Autodesk Fusion 360 part; units mm, degrees
(part 4 of 8)
  spline S105 degree 5 poles (194.1162, -114.5953) (194.0941, -114.6123) (193.999, -114.6851) (193.8315, -114.8142) (193.592, -115.0006) (193.2814, -115.2456) (192.9226, -115.5331) (192.5656, -115.8236) (192.2106, -116.117) (191.8576, -116.4134) (191.5064, -116.7127) (191.1571, -117.0147) (190.8096, -117.3193) (190.4637, -117.6264) (190.1196, -117.9359) (189.777, -118.2478) (189.4361, -118.562) (189.0968, -118.8784) (188.759, -119.1971) (188.4229, -119.5179) (188.0883, -119.841) (187.7552, -120.1661) (187.4236, -120.4933) (187.0935, -120.8225) (186.7649, -121.1538) (186.4377, -121.4869) (186.112, -121.822) (185.7877, -122.1589) (185.4648, -122.4977) (185.1433, -122.8384) (184.8232, -123.1808) (184.5045, -123.5251) (184.1871, -123.8711) (183.8711, -124.2188) (183.5565, -124.5682) (183.2431, -124.9194) (182.9312, -125.2722) (182.6205, -125.6266) (182.3112, -125.9826) (182.0031, -126.3403) (181.6964, -126.6995) (181.3909, -127.0603) (181.0867, -127.4227) (180.7838, -127.7866) (180.4822, -128.152) (180.1819, -128.5189) (179.8827, -128.8873) (179.5849, -129.2572) (179.2883, -129.6285) (178.9929, -130.0013) (178.6988, -130.3755) (178.4058, -130.7511) (178.1142, -131.1281) (177.8237, -131.5064) (177.5344, -131.8862) (177.2464, -132.2673) (176.9596, -132.6498) (176.6739, -133.0336) (176.3895, -133.4187) (176.1062, -133.8051) (175.8242, -134.1929) (175.5433, -134.5819) (175.3196, -134.8941) (175.1523, -135.1289) (175.041, -135.2857) (174.9854, -135.3641) knots 0.13851185 0.13851185 0.13851185 0.13851185 0.13851185 0.13851185 0.14285714 0.15714286 0.17142857 0.18571429 0.2 0.21428571 0.22857143 0.24285714 0.25714286 0.27142857 0.28571429 0.3 0.31428571 0.32857143 0.34285714 0.35714286 0.37142857 0.38571429 0.4 0.41428571 0.42857143 0.44285714 0.45714286 0.47142857 0.48571429 0.5 0.51428571 0.52857143 0.54285714 0.55714286 0.57142857 0.58571429 0.6 0.61428571 0.62857143 0.64285714 0.65714286 0.67142857 0.68571429 0.7 0.71428571 0.72857143 0.74285714 0.75714286 0.77142857 0.78571429 0.8 0.81428571 0.82857143 0.84285714 0.85714286 0.87142857 0.88571429 0.9 0.91428571 0.92857143 0.94285714 0.95714286 0.97142857 0.98571429 1 1 1 1 1 1
  arc A53 (174.9854, -135.3641) -> (179.8933, -143.8648) centre (452.3696, 19.1166) ccw
  spline S106 degree 5 poles (179.8933, -143.8648) (179.989, -143.8559) (180.1804, -143.8379) (180.4674, -143.8104) (180.8497, -143.7727) (181.327, -143.724) (181.8038, -143.6736) (182.2801, -143.6215) (182.7558, -143.5677) (183.231, -143.5123) (183.7057, -143.4551) (184.1797, -143.3962) (184.6533, -143.3356) (185.1262, -143.2732) (185.5985, -143.2091) (186.0702, -143.1433) (186.5414, -143.0756) (187.0119, -143.0062) (187.4818, -142.935) (187.951, -142.862) (188.4196, -142.7871) (188.8875, -142.7105) (189.3548, -142.6319) (189.8214, -142.5516) (190.2873, -142.4693) (190.7525, -142.3852) (191.217, -142.2992) (191.6807, -142.2112) (192.1438, -142.1214) (192.606, -142.0295) (193.0676, -141.9357) (193.5283, -141.84) (193.9882, -141.7422) (194.4474, -141.6424) (194.9057, -141.5406) (195.3632, -141.4367) (195.8198, -141.3307) (196.2756, -141.2226) (196.7304, -141.1123) (197.1844, -141) (197.6374, -140.8854) (198.0895, -140.7686) (198.5407, -140.6496) (198.9909, -140.5284) (199.44, -140.4048) (199.8881, -140.2789) (200.3352, -140.1507) (200.7812, -140.02) (201.226, -139.8868) (201.6697, -139.7512) (202.1122, -139.613) (202.5536, -139.4723) (202.9937, -139.329) (203.4326, -139.1831) (203.8702, -139.0344) (204.3064, -138.8829) (204.7411, -138.7284) (205.1743, -138.5708) (205.606, -138.4101) (206.036, -138.2462) (206.4644, -138.0792) (206.8318, -137.9327) (207.113, -137.8185) (207.3086, -137.738) (207.4192, -137.6921) (207.445, -137.6814) knots -1 -1 -1 -1 -1 -1 -0.98571429 -0.97142857 -0.95714286 -0.94285714 -0.92857143 -0.91428571 -0.9 -0.88571429 -0.87142857 -0.85714286 -0.84285714 -0.82857143 -0.81428571 -0.8 -0.78571429 -0.77142857 -0.75714286 -0.74285714 -0.72857143 -0.71428571 -0.7 -0.68571429 -0.67142857 -0.65714286 -0.64285714 -0.62857143 -0.61428571 -0.6 -0.58571429 -0.57142857 -0.55714286 -0.54285714 -0.52857143 -0.51428571 -0.5 -0.48571429 -0.47142857 -0.45714286 -0.44285714 -0.42857143 -0.41428571 -0.4 -0.38571429 -0.37142857 -0.35714286 -0.34285714 -0.32857143 -0.31428571 -0.3 -0.28571429 -0.27142857 -0.25714286 -0.24285714 -0.22857143 -0.21428571 -0.2 -0.18571429 -0.17142857 -0.15714286 -0.14285714 -0.13851185 -0.13851185 -0.13851185 -0.13851185 -0.13851185 -0.13851185
  spline S107 degree 3 poles (209.3868, -138.2841) (209.2745, -138.1106) (209.1293, -137.9607) (208.7896, -137.7251) (208.5983, -137.6415) (208.2383, -137.5621) (208.0756, -137.5516) (207.7528, -137.5802) (207.5946, -137.6192) (207.445, -137.6814) knots 0 0 0 0 0.062015 0.062015 0.12403 0.12403 0.172638 0.172638 0.221247 0.221247 0.221247 0.221247
  arc A54 (209.3868, -138.2841) -> (213.9648, -145.1355) centre (452.3696, 19.1166) ccw
  spline S108 degree 3 poles (213.7785, -147.1602) (213.9249, -147.0143) (214.0414, -146.8411) (214.2013, -146.4599) (214.2433, -146.2555) (214.2463, -145.8867) (214.2227, -145.7255) (214.1277, -145.4157) (214.0567, -145.2689) (213.9648, -145.1355) knots 0 0 0 0 0.062015 0.062015 0.12403 0.12403 0.172638 0.172638 0.221247 0.221247 0.221247 0.221247
  spline S109 degree 5 poles (213.7785, -147.1602) (213.7588, -147.18) (213.6741, -147.2645) (213.5248, -147.4144) (213.3117, -147.6305) (213.0357, -147.9139) (212.7175, -148.2458) (212.4015, -148.5804) (212.0879, -148.9177) (211.7765, -149.2576) (211.4674, -149.6001) (211.1605, -149.9451) (210.8557, -150.2925) (210.5529, -150.6421) (210.2521, -150.9939) (209.9532, -151.3478) (209.6562, -151.7038) (209.3611, -152.0618) (209.0678, -152.4219) (208.7764, -152.7839) (208.4868, -153.1478) (208.199, -153.5136) (207.913, -153.8813) (207.6287, -154.2508) (207.3461, -154.6221) (207.0652, -154.9951) (206.786, -155.3698) (206.5085, -155.7462) (206.2326, -156.1243) (205.9583, -156.504) (205.6856, -156.8853) (205.4145, -157.2682) (205.1451, -157.6526) (204.8772, -158.0386) (204.6108, -158.4262) (204.346, -158.8152) (204.0828, -159.2057) (203.821, -159.5976) (203.5608, -159.991) (203.3021, -160.3858) (203.0448, -160.782) (202.7891, -161.1796) (202.5348, -161.5786) (202.282, -161.9789) (202.0307, -162.3805) (201.7808, -162.7835) (201.5323, -163.1878) (201.2853, -163.5934) (201.0396, -164.0002) (200.7955, -164.4084) (200.5527, -164.8177) (200.3113, -165.2284) (200.0713, -165.6402) (199.8327, -166.0533) (199.5955, -166.4675) (199.3597, -166.883) (199.1252, -167.2996) (198.8921, -167.7174) (198.6604, -168.1364) (198.43, -168.5565) (198.201, -168.9777) (197.9733, -169.4) (197.7922, -169.7388) (197.657, -169.9934) (197.5671, -170.1634) (197.5222, -170.2484) knots 0.13851185 0.13851185 0.13851185 0.13851185 0.13851185 0.13851185 0.14285714 0.15714286 0.17142857 0.18571429 0.2 0.21428571 0.22857143 0.24285714 0.25714286 0.27142857 0.28571429 0.3 0.31428571 0.32857143 0.34285714 0.35714286 0.37142857 0.38571429 0.4 0.41428571 0.42857143 0.44285714 0.45714286 0.47142857 0.48571429 0.5 0.51428571 0.52857143 0.54285714 0.55714286 0.57142857 0.58571429 0.6 0.61428571 0.62857143 0.64285714 0.65714286 0.67142857 0.68571429 0.7 0.71428571 0.72857143 0.74285714 0.75714286 0.77142857 0.78571429 0.8 0.81428571 0.82857143 0.84285714 0.85714286 0.87142857 0.88571429 0.9 0.91428571 0.92857143 0.94285714 0.95714286 0.97142857 0.98571429 1 1 1 1 1 1
  arc A55 (197.5222, -170.2484) -> (203.4977, -178.0357) centre (452.3696, 19.1166) ccw
  spline S110 degree 5 poles (203.4977, -178.0357) (203.5914, -178.0144) (203.7789, -177.9716) (204.0598, -177.9069) (204.4339, -177.8197) (204.9008, -177.709) (205.3669, -177.5968) (205.8323, -177.483) (206.297, -177.3676) (206.7609, -177.2506) (207.224, -177.132) (207.6863, -177.0117) (208.1479, -176.8898) (208.6086, -176.7662) (209.0685, -176.641) (209.5276, -176.5141) (209.9859, -176.3856) (210.4433, -176.2553) (210.8999, -176.1234) (211.3556, -175.9898) (211.8104, -175.8544) (212.2643, -175.7173) (212.7173, -175.5785) (213.1695, -175.4379) (213.6206, -175.2955) (214.0709, -175.1514) (214.5202, -175.0055) (214.9685, -174.8578) (215.4158, -174.7082) (215.8621, -174.5568) (216.3075, -174.4036) (216.7518, -174.2485) (217.195, -174.0916) (217.6372, -173.9327) (218.0783, -173.7719) (218.5183, -173.6092) (218.9572, -173.4445) (219.3949, -173.2778) (219.8315, -173.1092) (220.2669, -172.9385) (220.7012, -172.7658) (221.1341, -172.591) (221.5659, -172.4141) (221.9964, -172.2352) (222.4256, -172.054) (222.8534, -171.8707) (223.2799, -171.6852) (223.705, -171.4974) (224.1287, -171.3073) (224.5509, -171.1149) (224.9716, -170.9202) (225.3908, -170.7231) (225.8085, -170.5236) (226.2246, -170.3216) (226.639, -170.1171) (227.0517, -169.9099) (227.4625, -169.7) (227.8715, -169.4872) (228.2784, -169.2716) (228.6834, -169.053) (229.0863, -168.8315) (229.4315, -168.6383) (229.6954, -168.4883) (229.8788, -168.3829) (229.9824, -168.323) (230.0066, -168.309) knots -1 -1 -1 -1 -1 -1 -0.98571429 -0.97142857 -0.95714286 -0.94285714 -0.92857143 -0.91428571 -0.9 -0.88571429 -0.87142857 -0.85714286 -0.84285714 -0.82857143 -0.81428571 -0.8 -0.78571429 -0.77142857 -0.75714286 -0.74285714 -0.72857143 -0.71428571 -0.7 -0.68571429 -0.67142857 -0.65714286 -0.64285714 -0.62857143 -0.61428571 -0.6 -0.58571429 -0.57142857 -0.55714286 -0.54285714 -0.52857143 -0.51428571 -0.5 -0.48571429 -0.47142857 -0.45714286 -0.44285714 -0.42857143 -0.41428571 -0.4 -0.38571429 -0.37142857 -0.35714286 -0.34285714 -0.32857143 -0.31428571 -0.3 -0.28571429 -0.27142857 -0.25714286 -0.24285714 -0.22857143 -0.21428571 -0.2 -0.18571429 -0.17142857 -0.15714286 -0.14285714 -0.13851185 -0.13851185 -0.13851185 -0.13851185 -0.13851185 -0.13851185
  spline S111 degree 3 poles (232.0105, -168.6531) (231.8764, -168.4958) (231.7129, -168.3662) (231.3454, -168.1768) (231.1449, -168.119) (230.7775, -168.0872) (230.6149, -168.098) (230.2986, -168.1686) (230.1468, -168.2278) (230.0066, -168.309) knots 0 0 0 0 0.062015 0.062015 0.12403 0.12403 0.172638 0.172638 0.221247 0.221247 0.221247 0.221247
  arc A56 (232.0105, -168.6531) -> (237.4436, -174.8484) centre (452.3696, 19.1166) ccw
  spline S112 degree 3 poles (237.5232, -176.8801) (237.6493, -176.7163) (237.7421, -176.5294) (237.851, -176.1305) (237.8659, -175.9224) (237.8207, -175.5564) (237.7763, -175.3996) (237.6417, -175.1049) (237.5521, -174.9687) (237.4436, -174.8484) knots 0 0 0 0 0.062015 0.062015 0.12403 0.12403 0.172638 0.172638 0.221247 0.221247 0.221247 0.221247
  spline S113 degree 5 poles (237.5232, -176.8801) (237.5062, -176.9022) (237.4332, -176.9971) (237.3048, -177.1652) (237.1217, -177.4073) (236.8851, -177.7243) (236.6129, -178.0949) (236.3433, -178.4678) (236.0764, -178.8431) (235.8121, -179.2208) (235.5503, -179.6007) (235.2911, -179.9829) (235.0342, -180.367) (234.7796, -180.7532) (234.5273, -181.1413) (234.2772, -181.5312) (234.0292, -181.9229) (233.7833, -182.3164) (233.5396, -182.7116) (233.2979, -183.1085) (233.0583, -183.5071) (232.8207, -183.9074) (232.5851, -184.3093) (232.3515, -184.7127) (232.1198, -185.1177) (231.89, -185.5242) (231.6621, -185.9321) (231.436, -186.3415) (231.2118, -186.7524) (230.9894, -187.1646) (230.7689, -187.5783) (230.5501, -187.9933) (230.3331, -188.4096) (230.1179, -188.8273) (229.9044, -189.2463) (229.6927, -189.6665) (229.4826, -190.088) (229.2743, -190.5108) (229.0676, -190.9347) (228.8626, -191.3599) (228.6593, -191.7863) (228.4577, -192.2139) (228.2576, -192.6427) (228.0592, -193.0726) (227.8625, -193.5036) (227.6673, -193.9357) (227.4737, -194.369) (227.2818, -194.8033) (227.0914, -195.2388) (226.9025, -195.6753) (226.7152, -196.1129) (226.5295, -196.5515) (226.3454, -196.9911) (226.1627, -197.4318) (225.9816, -197.8735) (225.802, -198.3162) (225.624, -198.7598) (225.4474, -199.2045) (225.2723, -199.6501) (225.0987, -200.0967) (224.9266, -200.5442) (224.756, -200.9926) (224.6207, -201.3522) (224.5199, -201.6222) (224.453, -201.8024) (224.4196, -201.8926) knots 0.13851185 0.13851185 0.13851185 0.13851185 0.13851185 0.13851185 0.14285714 0.15714286 0.17142857 0.18571429 0.2 0.21428571 0.22857143 0.24285714 0.25714286 0.27142857 0.28571429 0.3 0.31428571 0.32857143 0.34285714 0.35714286 0.37142857 0.38571429 0.4 0.41428571 0.42857143 0.44285714 0.45714286 0.47142857 0.48571429 0.5 0.51428571 0.52857143 0.54285714 0.55714286 0.57142857 0.58571429 0.6 0.61428571 0.62857143 0.64285714 0.65714286 0.67142857 0.68571429 0.7 0.71428571 0.72857143 0.74285714 0.75714286 0.77142857 0.78571429 0.8 0.81428571 0.82857143 0.84285714 0.85714286 0.87142857 0.88571429 0.9 0.91428571 0.92857143 0.94285714 0.95714286 0.97142857 0.98571429 1 1 1 1 1 1
  arc A57 (224.4196, -201.8926) -> (231.3604, -208.8334) centre (452.3696, 19.1166) ccw
  spline S114 degree 5 poles (231.3604, -208.8334) (231.4505, -208.8) (231.6307, -208.7331) (231.9008, -208.6323) (232.2603, -208.4969) (232.7088, -208.3263) (233.1563, -208.1542) (233.6029, -207.9807) (234.0485, -207.8056) (234.4931, -207.629) (234.9368, -207.4509) (235.3795, -207.2713) (235.8212, -207.0902) (236.2619, -206.9076) (236.7015, -206.7234) (237.1401, -206.5377) (237.5777, -206.3504) (238.0142, -206.1616) (238.4496, -205.9712) (238.884, -205.7792) (239.3172, -205.5857) (239.7494, -205.3905) (240.1804, -205.1937) (240.6103, -204.9953) (241.039, -204.7953) (241.4666, -204.5936) (241.893, -204.3903) (242.3182, -204.1853) (242.7422, -203.9787) (243.165, -203.7704) (243.5865, -203.5603) (244.0067, -203.3486) (244.4257, -203.1351) (244.8433, -202.9198) (245.2597, -202.7029) (245.6747, -202.4841) (246.0883, -202.2635) (246.5006, -202.0412) (246.9114, -201.817) (247.3208, -201.5909) (247.7288, -201.363) (248.1353, -201.1332) (248.5402, -200.9015) (248.9437, -200.6678) (249.3456, -200.4323) (249.7458, -200.1947) (250.1445, -199.9551) (250.5414, -199.7134) (250.9366, -199.4696) (251.3301, -199.2238) (251.7218, -198.9758) (252.1117, -198.7256) (252.4997, -198.4733) (252.8859, -198.2188) (253.2701, -197.9619) (253.6522, -197.7027) (254.0322, -197.4409) (254.4098, -197.1766) (254.7851, -196.9096) (255.1581, -196.6401) (255.5287, -196.3678) (255.8457, -196.1313) (256.0877, -195.9482) (256.2558, -195.8197) (256.3507, -195.7468) (256.3729, -195.7298) knots -1 -1 -1 -1 -1 -1 -0.98571429 -0.97142857 -0.95714286 -0.94285714 -0.92857143 -0.91428571 -0.9 -0.88571429 -0.87142857 -0.85714286 -0.84285714 -0.82857143 -0.81428571 -0.8 -0.78571429 -0.77142857 -0.75714286 -0.74285714 -0.72857143 -0.71428571 -0.7 -0.68571429 -0.67142857 -0.65714286 -0.64285714 -0.62857143 -0.61428571 -0.6 -0.58571429 -0.57142857 -0.55714286 -0.54285714 -0.52857143 -0.51428571 -0.5 -0.48571429 -0.47142857 -0.45714286 -0.44285714 -0.42857143 -0.41428571 -0.4 -0.38571429 -0.37142857 -0.35714286 -0.34285714 -0.32857143 -0.31428571 -0.3 -0.28571429 -0.27142857 -0.25714286 -0.24285714 -0.22857143 -0.21428571 -0.2 -0.18571429 -0.17142857 -0.15714286 -0.14285714 -0.13851185 -0.13851185 -0.13851185 -0.13851185 -0.13851185 -0.13851185
  spline S115 degree 3 poles (258.4046, -195.8094) (258.2511, -195.6709) (258.0721, -195.5637) (257.683, -195.424) (257.4766, -195.3928) (257.1083, -195.4092) (256.9484, -195.4412) (256.6441, -195.5524) (256.5013, -195.631) (256.3729, -195.7298) knots 0 0 0 0 0.062015 0.062015 0.12403 0.12403 0.172638 0.172638 0.221247 0.221247 0.221247 0.221247
  arc A58 (258.4046, -195.8094) -> (264.5998, -201.2425) centre (452.3696, 19.1166) ccw
  spline S116 degree 3 poles (264.9439, -203.2464) (265.0475, -203.0675) (265.1152, -202.8701) (265.1711, -202.4605) (265.1587, -202.2522) (265.0661, -201.8952) (265.0017, -201.7455) (264.8297, -201.4709) (264.7232, -201.3475) (264.5998, -201.2425) knots 0 0 0 0 0.062015 0.062015 0.12403 0.12403 0.172638 0.172638 0.221247 0.221247 0.221247 0.221247
  spline S117 degree 5 poles (264.9439, -203.2464) (264.9299, -203.2706) (264.87, -203.3742) (264.7646, -203.5576) (264.6147, -203.8215) (264.4215, -204.1666) (264.2, -204.5696) (263.9814, -204.9746) (263.7657, -205.3815) (263.553, -205.7904) (263.343, -206.2013) (263.1359, -206.614) (262.9314, -207.0284) (262.7294, -207.4445) (262.5299, -207.8622) (262.3328, -208.2814) (262.138, -208.7021) (261.9456, -209.1243) (261.7555, -209.5479) (261.5678, -209.973) (261.3822, -210.3995) (261.1989, -210.8274) (261.0178, -211.2566) (260.8388, -211.6871) (260.662, -212.1188) (260.4872, -212.5518) (260.3145, -212.986) (260.1438, -213.4214) (259.9751, -213.858) (259.8085, -214.2958) (259.6438, -214.7347) (259.4811, -215.1747) (259.3203, -215.6158) (259.1614, -216.058) (259.0044, -216.5012) (258.8493, -216.9455) (258.6961, -217.3908) (258.5447, -217.8372) (258.3952, -218.2845) (258.2475, -218.7328) (258.1016, -219.1821) (257.9574, -219.6323) (257.8151, -220.0835) (257.6745, -220.5356) (257.5357, -220.9886) (257.3986, -221.4426) (257.2632, -221.8974) (257.1296, -222.3531) (256.9976, -222.8097) (256.8674, -223.2671) (256.7388, -223.7253) (256.612, -224.1844) (256.4867, -224.6444) (256.3632, -225.1051) (256.2413, -225.5666) (256.121, -226.029) (256.0024, -226.4921) (255.8854, -226.956) (255.7699, -227.4206) (255.6561, -227.8861) (255.5439, -228.3522) (255.4333, -228.8191) (255.3461, -229.1932) (255.2814, -229.4741) (255.2386, -229.6615) (255.2172, -229.7553) knots 0.13851185 0.13851185 0.13851185 0.13851185 0.13851185 0.13851185 0.14285714 0.15714286 0.17142857 0.18571429 0.2 0.21428571 0.22857143 0.24285714 0.25714286 0.27142857 0.28571429 0.3 0.31428571 0.32857143 0.34285714 0.35714286 0.37142857 0.38571429 0.4 0.41428571 0.42857143 0.44285714 0.45714286 0.47142857 0.48571429 0.5 0.51428571 0.52857143 0.54285714 0.55714286 0.57142857 0.58571429 0.6 0.61428571 0.62857143 0.64285714 0.65714286 0.67142857 0.68571429 0.7 0.71428571 0.72857143 0.74285714 0.75714286 0.77142857 0.78571429 0.8 0.81428571 0.82857143 0.84285714 0.85714286 0.87142857 0.88571429 0.9 0.91428571 0.92857143 0.94285714 0.95714286 0.97142857 0.98571429 1 1 1 1 1 1
  arc A59 (255.2172, -229.7553) -> (263.0046, -235.7307) centre (452.3696, 19.1166) ccw
  spline S118 degree 5 poles (263.0046, -235.7307) (263.0896, -235.6859) (263.2595, -235.596) (263.5141, -235.4608) (263.8529, -235.2797) (264.2753, -235.052) (264.6965, -234.823) (265.1166, -234.5926) (265.5355, -234.3608) (265.9533, -234.1277) (266.37, -233.8933) (266.7854, -233.6575) (267.1997, -233.4202) (267.6128, -233.1817) (268.0246, -232.9417) (268.4352, -232.7003) (268.8446, -232.4575) (269.2527, -232.2133) (269.6596, -231.9677) (270.0652, -231.7207) (270.4695, -231.4722) (270.8724, -231.2223) (271.2741, -230.971) (271.6744, -230.7181) (272.0734, -230.4639) (272.471, -230.2081) (272.8672, -229.9509) (273.262, -229.6922) (273.6554, -229.4319) (274.0473, -229.1702) (274.4378, -228.9069) (274.8268, -228.6421) (275.2143, -228.3758) (275.6003, -228.1079) (275.9848, -227.8384) (276.3677, -227.5674) (276.749, -227.2947) (277.1287, -227.0204) (277.5068, -226.7445) (277.8832, -226.4669) (278.2579, -226.1877) (278.6309, -225.9068) (279.0021, -225.6243) (279.3716, -225.34) (279.7393, -225.0539) (280.1052, -224.7661) (280.4691, -224.4766) (280.8311, -224.1851) (281.1911, -223.8919) (281.5491, -223.5968) (281.9051, -223.2998) (282.259, -223.0009) (282.6108, -222.7001) (282.9605, -222.3973) (283.3079, -222.0925) (283.6529, -221.7856) (283.9954, -221.4765) (284.3353, -221.1651) (284.6726, -220.8515) (285.0071, -220.5355) (285.3391, -220.2172) (285.6225, -219.9413) (285.8385, -219.7282) (285.9884, -219.5789) (286.073, -219.4942) (286.0927, -219.4744) knots -1 -1 -1 -1 -1 -1 -0.98571429 -0.97142857 -0.95714286 -0.94285714 -0.92857143 -0.91428571 -0.9 -0.88571429 -0.87142857 -0.85714286 -0.84285714 -0.82857143 -0.81428571 -0.8 -0.78571429 -0.77142857 -0.75714286 -0.74285714 -0.72857143 -0.71428571 -0.7 -0.68571429 -0.67142857 -0.65714286 -0.64285714 -0.62857143 -0.61428571 -0.6 -0.58571429 -0.57142857 -0.55714286 -0.54285714 -0.52857143 -0.51428571 -0.5 -0.48571429 -0.47142857 -0.45714286 -0.44285714 -0.42857143 -0.41428571 -0.4 -0.38571429 -0.37142857 -0.35714286 -0.34285714 -0.32857143 -0.31428571 -0.3 -0.28571429 -0.27142857 -0.25714286 -0.24285714 -0.22857143 -0.21428571 -0.2 -0.18571429 -0.17142857 -0.15714286 -0.14285714 -0.13851185 -0.13851185 -0.13851185 -0.13851185 -0.13851185 -0.13851185
  spline S119 degree 3 poles (288.1174, -219.2882) (287.9472, -219.1709) (287.7557, -219.088) (287.3517, -219.0002) (287.1431, -218.9962) (286.78, -219.0606) (286.6257, -219.1132) (286.3384, -219.2632) (286.2071, -219.3597) (286.0927, -219.4744) knots 0 0 0 0 0.062015 0.062015 0.12403 0.12403 0.172638 0.172638 0.221247 0.221247 0.221247 0.221247
  arc A60 (288.1174, -219.2882) -> (294.9688, -223.8661) centre (452.3696, 19.1166) ccw
  spline S120 degree 3 poles (295.5716, -225.808) (295.6509, -225.6171) (295.6923, -225.4126) (295.6942, -224.9992) (295.6548, -224.7942) (295.5164, -224.4524) (295.4329, -224.3125) (295.2265, -224.0626) (295.1048, -223.9542) (294.9688, -223.8661) knots 0 0 0 0 0.062015 0.062015 0.12403 0.12403 0.172638 0.172638 0.221247 0.221247 0.221247 0.221247
  spline S121 degree 5 poles (295.5716, -225.808) (295.5609, -225.8338) (295.515, -225.9443) (295.4344, -226.14) (295.3202, -226.4211) (295.1737, -226.7886) (295.0067, -227.217) (294.8429, -227.647) (294.6821, -228.0786) (294.5246, -228.5118) (294.3701, -228.9466) (294.2186, -229.3828) (294.0699, -229.8203) (293.924, -230.2592) (293.7807, -230.6994) (293.64, -231.1407) (293.5018, -231.5833) (293.3661, -232.027) (293.233, -232.4718) (293.1023, -232.9178) (292.974, -233.3648) (292.8481, -233.813) (292.7246, -234.2621) (292.6033, -234.7123) (292.4843, -235.1634) (292.3676, -235.6155) (292.253, -236.0686) (292.1406, -236.5225) (292.0304, -236.9774) (291.9223, -237.4332) (291.8163, -237.8898) (291.7124, -238.3473) (291.6106, -238.8056) (291.5108, -239.2647) (291.413, -239.7247) (291.3172, -240.1854) (291.2234, -240.6469) (291.1316, -241.1092) (291.0417, -241.5722) (290.9538, -242.036) (290.8678, -242.5005) (290.7836, -242.9657) (290.7014, -243.4316) (290.621, -243.8982) (290.5425, -244.3654) (290.4658, -244.8334) (290.391, -245.302) (290.318, -245.7712) (290.2468, -246.2411) (290.1774, -246.7116) (290.1097, -247.1827) (290.0438, -247.6545) (289.9797, -248.1268) (289.9174, -248.5997) (289.8568, -249.0732) (289.7979, -249.5473) (289.7407, -250.0219) (289.6852, -250.4971) (289.6314, -250.9729) (289.5794, -251.4492) (289.529, -251.926) (289.4802, -252.4033) (289.4426, -252.7856) (289.4151, -253.0726) (289.3971, -253.264) (289.3882, -253.3597) knots 0.13851185 0.13851185 0.13851185 0.13851185 0.13851185 0.13851185 0.14285714 0.15714286 0.17142857 0.18571429 0.2 0.21428571 0.22857143 0.24285714 0.25714286 0.27142857 0.28571429 0.3 0.31428571 0.32857143 0.34285714 0.35714286 0.37142857 0.38571429 0.4 0.41428571 0.42857143 0.44285714 0.45714286 0.47142857 0.48571429 0.5 0.51428571 0.52857143 0.54285714 0.55714286 0.57142857 0.58571429 0.6 0.61428571 0.62857143 0.64285714 0.65714286 0.67142857 0.68571429 0.7 0.71428571 0.72857143 0.74285714 0.75714286 0.77142857 0.78571429 0.8 0.81428571 0.82857143 0.84285714 0.85714286 0.87142857 0.88571429 0.9 0.91428571 0.92857143 0.94285714 0.95714286 0.97142857 0.98571429 1 1 1 1 1 1
  arc A61 (289.3882, -253.3597) -> (297.8889, -258.2676) centre (452.3696, 19.1166) ccw
  spline S122 degree 5 poles (297.8889, -258.2676) (297.9673, -258.212) (298.1241, -258.1007) (298.3588, -257.9334) (298.6711, -257.7097) (299.0601, -257.4288) (299.4478, -257.1467) (299.8343, -256.8635) (300.2194, -256.579) (300.6032, -256.2934) (300.9856, -256.0066) (301.3668, -255.7185) (301.7465, -255.4293) (302.1249, -255.1388) (302.5019, -254.8471) (302.8775, -254.5542) (303.2517, -254.2601) (303.6245, -253.9647) (303.9958, -253.6681) (304.3656, -253.3702) (304.734, -253.0711) (305.1009, -252.7707) (305.4664, -252.4691) (305.8303, -252.1662) (306.1926, -251.8621) (306.5534, -251.5566) (306.9127, -251.2498) (307.2703, -250.9418) (307.6264, -250.6325) (307.9808, -250.3218) (308.3336, -250.0098) (308.6847, -249.6965) (309.0342, -249.3819) (309.3819, -249.0659) (309.7279, -248.7485) (310.0721, -248.4298) (310.4146, -248.1097) (310.7552, -247.7882) (311.094, -247.4653) (311.431, -247.141) (311.7661, -246.8153) (312.0992, -246.4881) (312.4304, -246.1595) (312.7596, -245.8294) (313.0869, -245.4978) (313.412, -245.1647) (313.735, -244.8301) (314.0559, -244.4939) (314.3746, -244.1562) (314.691, -243.8169) (315.0051, -243.4759) (315.317, -243.1334) (315.6266, -242.7892) (315.9337, -242.4434) (316.2383, -242.0959) (316.5403, -241.7465) (316.8396, -241.3954) (317.1359, -241.0423) (317.4294, -240.6873) (317.7198, -240.3304) (318.0074, -239.9716) (318.2523, -239.661) (318.4387, -239.4215) (318.5679, -239.2539) (318.6407, -239.1589) (318.6576, -239.1367) knots -1 -1 -1 -1 -1 -1 -0.98571429 -0.97142857 -0.95714286 -0.94285714 -0.92857143 -0.91428571 -0.9 -0.88571429 -0.87142857 -0.85714286 -0.84285714 -0.82857143 -0.81428571 -0.8 -0.78571429 -0.77142857 -0.75714286 -0.74285714 -0.72857143 -0.71428571 -0.7 -0.68571429 -0.67142857 -0.65714286 -0.64285714 -0.62857143 -0.61428571 -0.6 -0.58571429 -0.57142857 -0.55714286 -0.54285714 -0.52857143 -0.51428571 -0.5 -0.48571429 -0.47142857 -0.45714286 -0.44285714 -0.42857143 -0.41428571 -0.4 -0.38571429 -0.37142857 -0.35714286 -0.34285714 -0.32857143 -0.31428571 -0.3 -0.28571429 -0.27142857 -0.25714286 -0.24285714 -0.22857143 -0.21428571 -0.2 -0.18571429 -0.17142857 -0.15714286 -0.14285714 -0.13851185 -0.13851185 -0.13851185 -0.13851185 -0.13851185 -0.13851185
  spline S123 degree 3 poles (320.6407, -238.6878) (320.4566, -238.5937) (320.2559, -238.5365) (319.8439, -238.5023) (319.6366, -238.5255) (319.285, -238.6368) (319.1389, -238.709) (318.8737, -238.8952) (318.7561, -239.0081) (318.6576, -239.1367) knots 0 0 0 0 0.062015 0.062015 0.12403 0.12403 0.172638 0.172638 0.221247 0.221247 0.221247 0.221247
  arc A62 (320.6407, -238.6878) -> (328.031, -242.3323) centre (452.3696, 19.1166) ccw
  spline S124 degree 3 poles (328.8821, -244.1789) (328.9359, -243.9793) (328.9501, -243.7711) (328.8981, -243.3609) (328.8322, -243.1629) (328.6504, -242.8421) (328.5494, -242.7142) (328.3122, -242.4935) (328.1774, -242.4019) (328.031, -242.3323) knots 0 0 0 0 0.062015 0.062015 0.12403 0.12403 0.172638 0.172638 0.221247 0.221247 0.221247 0.221247
  spline S125 degree 5 poles (328.8821, -244.1789) (328.8748, -244.2058) (328.8438, -244.3214) (328.7894, -244.5259) (328.7129, -244.8196) (328.6156, -245.203) (328.506, -245.6495) (328.3996, -246.0973) (328.2966, -246.5462) (328.1969, -246.9962) (328.1005, -247.4474) (328.0072, -247.8997) (327.9169, -248.3529) (327.8296, -248.8071) (327.7449, -249.2622) (327.663, -249.7181) (327.5838, -250.1749) (327.5073, -250.6325) (327.4333, -251.0909) (327.3619, -251.5501) (327.2931, -252.0101) (327.2268, -252.4708) (327.1629, -252.9323) (327.1015, -253.3944) (327.0424, -253.8572) (326.9856, -254.3207) (326.9312, -254.7848) (326.879, -255.2496) (326.8291, -255.7149) (326.7814, -256.1809) (326.7359, -256.6475) (326.6926, -257.1146) (326.6515, -257.5823) (326.6125, -258.0505) (326.5756, -258.5193) (326.5408, -258.9886) (326.508, -259.4584) (326.4773, -259.9287) (326.4486, -260.3995) (326.422, -260.8708) (326.3973, -261.3425) (326.3746, -261.8147) (326.3539, -262.2874) (326.3351, -262.7605) (326.3183, -263.234) (326.3033, -263.7079) (326.2903, -264.1823) (326.2792, -264.657) (326.2699, -265.1322) (326.2625, -265.6077) (326.2569, -266.0837) (326.2532, -266.5599) (326.2513, -267.0366) (326.2512, -267.5136) (326.2529, -267.991) (326.2564, -268.4687) (326.2616, -268.9468) (326.2687, -269.4251) (326.2774, -269.9038) (326.288, -270.3828) (326.3002, -270.8621) (326.3142, -271.3417) (326.3268, -271.7257) (326.337, -272.0138) (326.3441, -272.2059) (326.3478, -272.302) knots 0.13851185 0.13851185 0.13851185 0.13851185 0.13851185 0.13851185 0.14285714 0.15714286 0.17142857 0.18571429 0.2 0.21428571 0.22857143 0.24285714 0.25714286 0.27142857 0.28571429 0.3 0.31428571 0.32857143 0.34285714 0.35714286 0.37142857 0.38571429 0.4 0.41428571 0.42857143 0.44285714 0.45714286 0.47142857 0.48571429 0.5 0.51428571 0.52857143 0.54285714 0.55714286 0.57142857 0.58571429 0.6 0.61428571 0.62857143 0.64285714 0.65714286 0.67142857 0.68571429 0.7 0.71428571 0.72857143 0.74285714 0.75714286 0.77142857 0.78571429 0.8 0.81428571 0.82857143 0.84285714 0.85714286 0.87142857 0.88571429 0.9 0.91428571 0.92857143 0.94285714 0.95714286 0.97142857 0.98571429 1 1 1 1 1 1
  arc A63 (326.3478, -272.302) -> (335.4164, -276.0583) centre (452.3696, 19.1166) ccw
  spline S126 degree 5 poles (335.4164, -276.0583) (335.4869, -275.9929) (335.6278, -275.8621) (335.8387, -275.6656) (336.1191, -275.403) (336.4681, -275.0738) (336.8157, -274.7435) (337.1618, -274.4123) (337.5065, -274.08) (337.8498, -273.7467) (338.1915, -273.4124) (338.5318, -273.0771) (338.8705, -272.7407) (339.2078, -272.4034) (339.5435, -272.065) (339.8776, -271.7255) (340.2102, -271.3851) (340.5412, -271.0436) (340.8707, -270.701) (341.1985, -270.3574) (341.5247, -270.0128) (341.8493, -269.6671) (342.1722, -269.3204) (342.4934, -268.9726) (342.813, -268.6237) (343.1309, -268.2738) (343.447, -267.9228) (343.7614, -267.5707) (344.074, -267.2175) (344.3848, -266.8632) (344.6939, -266.5079) (345.0011, -266.1514) (345.3065, -265.7938) (345.61, -265.4352) (345.9116, -265.0754) (346.2113, -264.7144) (346.5091, -264.3524) (346.8048, -263.9892) (347.0986, -263.6248) (347.3903, -263.2593) (347.68, -262.8926) (347.9676, -262.5247) (348.2531, -262.1557) (348.5364, -261.7855) (348.8175, -261.414) (349.0964, -261.0413) (349.373, -260.6674) (349.6473, -260.2923) (349.9191, -259.9158) (350.1885, -259.5381) (350.4555, -259.1591) (350.72, -258.7788) (350.982, -258.3971) (351.2413, -258.0142) (351.498, -257.6298) (351.7518, -257.2441) (352.0027, -256.8569) (352.2504, -256.4682) (352.495, -256.0779) (352.7364, -255.6861) (352.9746, -255.2928) (353.177, -254.9529) (353.3305, -254.6911) (353.4367, -254.5082) (353.4964, -254.4044) (353.5104, -254.3803) knots -1 -1 -1 -1 -1 -1 -0.98571429 -0.97142857 -0.95714286 -0.94285714 -0.92857143 -0.91428571 -0.9 -0.88571429 -0.87142857 -0.85714286 -0.84285714 -0.82857143 -0.81428571 -0.8 -0.78571429 -0.77142857 -0.75714286 -0.74285714 -0.72857143 -0.71428571 -0.7 -0.68571429 -0.67142857 -0.65714286 -0.64285714 -0.62857143 -0.61428571 -0.6 -0.58571429 -0.57142857 -0.55714286 -0.54285714 -0.52857143 -0.51428571 -0.5 -0.48571429 -0.47142857 -0.45714286 -0.44285714 -0.42857143 -0.41428571 -0.4 -0.38571429 -0.37142857 -0.35714286 -0.34285714 -0.32857143 -0.31428571 -0.3 -0.28571429 -0.27142857 -0.25714286 -0.24285714 -0.22857143 -0.21428571 -0.2 -0.18571429 -0.17142857 -0.15714286 -0.14285714 -0.13851185 -0.13851185 -0.13851185 -0.13851185 -0.13851185 -0.13851185
  spline S127 degree 3 poles (355.4179, -253.6763) (355.2231, -253.6071) (355.0167, -253.5765) (354.6037, -253.5964) (354.4011, -253.6465) (354.0671, -253.8027) (353.9317, -253.8934) (353.693, -254.1126) (353.5912, -254.2398) (353.5104, -254.3803) knots 0 0 0 0 0.062015 0.062015 0.12403 0.12403 0.172638 0.172638 0.221247 0.221247 0.221247 0.221247
  arc A64 (355.4179, -253.6763) -> (363.2207, -256.325) centre (452.3696, 19.1166) ccw
  spline S128 degree 3 poles (364.3055, -258.0447) (364.3328, -257.8398) (364.3197, -257.6315) (364.2146, -257.2317) (364.1235, -257.0439) (363.9013, -256.7496) (363.7845, -256.636) (363.5205, -256.4481) (363.3749, -256.3749) (363.2207, -256.325) knots 0 0 0 0 0.062015 0.062015 0.12403 0.12403 0.172638 0.172638 0.221247 0.221247 0.221247 0.221247
  spline S129 degree 5 poles (364.3055, -258.0447) (364.3018, -258.0724) (364.2861, -258.191) (364.2589, -258.4008) (364.2214, -258.702) (364.175, -259.0948) (364.1246, -259.5519) (364.0776, -260.0097) (364.034, -260.4682) (363.994, -260.9274) (363.9572, -261.3873) (363.9238, -261.8478) (363.8934, -262.309) (363.8661, -262.7707) (363.8416, -263.2329) (363.8199, -263.6957) (363.801, -264.1589) (363.7848, -264.6226) (363.7713, -265.0867) (363.7605, -265.5513) (363.7523, -266.0163) (363.7467, -266.4818) (363.7436, -266.9476) (363.743, -267.4138) (363.7448, -267.8804) (363.749, -268.3473) (363.7556, -268.8146) (363.7646, -269.2821) (363.7758, -269.75) (363.7894, -270.2182) (363.8052, -270.6867) (363.8232, -271.1555) (363.8435, -271.6246) (363.8659, -272.0939) (363.8905, -272.5635) (363.9172, -273.0333) (363.9461, -273.5034) (363.977, -273.9737) (364.0101, -274.4442) (364.0452, -274.9149) (364.0823, -275.3858) (364.1214, -275.8569) (364.1626, -276.3283) (364.2057, -276.7998) (364.2508, -277.2714) (364.2979, -277.7433) (364.3469, -278.2153) (364.3978, -278.6874) (364.4506, -279.1597) (364.5053, -279.6322) (364.5619, -280.1047) (364.6204, -280.5774) (364.6807, -281.0503) (364.7429, -281.5232) (364.8069, -281.9963) (364.8727, -282.4695) (364.9403, -282.9427) (365.0097, -283.4161) (365.0809, -283.8895) (365.1539, -284.3631) (365.2286, -284.8367) (365.3051, -285.3104) (365.3676, -285.6894) (365.4154, -285.9737) (365.4475, -286.1632) (365.4637, -286.258) knots 0.13851185 0.13851185 0.13851185 0.13851185 0.13851185 0.13851185 0.14285714 0.15714286 0.17142857 0.18571429 0.2 0.21428571 0.22857143 0.24285714 0.25714286 0.27142857 0.28571429 0.3 0.31428571 0.32857143 0.34285714 0.35714286 0.37142857 0.38571429 0.4 0.41428571 0.42857143 0.44285714 0.45714286 0.47142857 0.48571429 0.5 0.51428571 0.52857143 0.54285714 0.55714286 0.57142857 0.58571429 0.6 0.61428571 0.62857143 0.64285714 0.65714286 0.67142857 0.68571429 0.7 0.71428571 0.72857143 0.74285714 0.75714286 0.77142857 0.78571429 0.8 0.81428571 0.82857143 0.84285714 0.85714286 0.87142857 0.88571429 0.9 0.91428571 0.92857143 0.94285714 0.95714286 0.97142857 0.98571429 1 1 1 1 1 1
  arc A65 (365.4637, -286.258) -> (374.945, -288.7985) centre (452.3696, 19.1166) ccw
  spline S130 degree 5 poles (374.945, -288.7985) (375.0063, -288.7245) (375.129, -288.5764) (375.3124, -288.3541) (375.5561, -288.0571) (375.8592, -287.6851) (376.1607, -287.3123) (376.4607, -286.9387) (376.759, -286.5643) (377.0558, -286.1891) (377.351, -285.813) (377.6446, -285.4361) (377.9366, -285.0585) (378.2269, -284.68) (378.5155, -284.3006) (378.8025, -283.9205) (379.0878, -283.5395) (379.3715, -283.1577) (379.6534, -282.7751) (379.9335, -282.3917) (380.212, -282.0074) (380.4886, -281.6223) (380.7635, -281.2364) (381.0366, -280.8496) (381.3079, -280.4621) (381.5774, -280.0736) (381.845, -279.6843) (382.1107, -279.2942) (382.3746, -278.9033) (382.6365, -278.5115) (382.8965, -278.1188) (383.1546, -277.7253) (383.4107, -277.3309) (383.6648, -276.9357) (383.9169, -276.5396) (384.1669, -276.1427) (384.4148, -275.7448) (384.6607, -275.3461) (384.9044, -274.9465) (385.1459, -274.5461) (385.3852, -274.1447) (385.6224, -273.7425) (385.8572, -273.3393) (386.0898, -272.9353) (386.32, -272.5303) (386.5479, -272.1244) (386.7733, -271.7176) (386.9962, -271.3098) (387.2166, -270.9011) (387.4344, -270.4915) (387.6497, -270.0808) (387.8623, -269.6693) (388.0722, -269.2567) (388.2793, -268.8432) (388.4836, -268.4286) (388.6849, -268.013) (388.8831, -267.5964) (389.078, -267.1787) (389.2695, -266.7598) (389.4577, -266.3399) (389.6426, -265.9188) (389.7988, -265.5554) (389.9169, -265.2759) (389.9982, -265.0806) (390.044, -264.97) (390.0546, -264.9442) knots -1 -1 -1 -1 -1 -1 -0.98571429 -0.97142857 -0.95714286 -0.94285714 -0.92857143 -0.91428571 -0.9 -0.88571429 -0.87142857 -0.85714286 -0.84285714 -0.82857143 -0.81428571 -0.8 -0.78571429 -0.77142857 -0.75714286 -0.74285714 -0.72857143 -0.71428571 -0.7 -0.68571429 -0.67142857 -0.65714286 -0.64285714 -0.62857143 -0.61428571 -0.6 -0.58571429 -0.57142857 -0.55714286 -0.54285714 -0.52857143 -0.51428571 -0.5 -0.48571429 -0.47142857 -0.45714286 -0.44285714 -0.42857143 -0.41428571 -0.4 -0.38571429 -0.37142857 -0.35714286 -0.34285714 -0.32857143 -0.31428571 -0.3 -0.28571429 -0.27142857 -0.25714286 -0.24285714 -0.22857143 -0.21428571 -0.2 -0.18571429 -0.17142857 -0.15714286 -0.14285714 -0.13851185 -0.13851185 -0.13851185 -0.13851185 -0.13851185 -0.13851185
  spline S131 degree 3 poles (391.8539, -263.9972) (391.6518, -263.954) (391.4431, -263.9507) (391.0363, -264.0243) (390.842, -264.1004) (390.5312, -264.2989) (390.4088, -264.4065) (390.2008, -264.6549) (390.1164, -264.7944) (390.0546, -264.9442) knots 0 0 0 0 0.062015 0.062015 0.12403 0.12403 0.172638 0.172638 0.221247 0.221247 0.221247 0.221247
  arc A66 (391.8539, -263.9972) -> (399.9357, -265.6048) centre (452.3696, 19.1166) ccw
  spline S132 degree 3 poles (401.2357, -267.1682) (401.236, -266.9615) (401.1959, -266.7567) (401.0394, -266.374) (400.9246, -266.1998) (400.6659, -265.937) (400.5353, -265.8396) (400.249, -265.6877) (400.0951, -265.6341) (399.9357, -265.6048) knots 0 0 0 0 0.062015 0.062015 0.12403 0.12403 0.172638 0.172638 0.221247 0.221247 0.221247 0.221247
  spline S133 degree 5 poles (401.2357, -267.1682) (401.2357, -267.1961) (401.2356, -267.3158) (401.236, -267.5274) (401.2381, -267.8309) (401.2434, -268.2264) (401.253, -268.6861) (401.2662, -269.1461) (401.2829, -269.6064) (401.3031, -270.0669) (401.3267, -270.5277) (401.3537, -270.9886) (401.3838, -271.4498) (401.4169, -271.9111) (401.453, -272.3726) (401.4919, -272.8342) (401.5336, -273.2959) (401.578, -273.7578) (401.6252, -274.2197) (401.6752, -274.6817) (401.7277, -275.1439) (401.7829, -275.606) (401.8407, -276.0683) (401.9009, -276.5306) (401.9636, -276.9929) (402.0288, -277.4553) (402.0963, -277.9177) (402.1662, -278.3801) (402.2384, -278.8425) (402.3129, -279.305) (402.3898, -279.7674) (402.4689, -280.2298) (402.5502, -280.6922) (402.6337, -281.1546) (402.7194, -281.617) (402.8072, -282.0793) (402.8971, -282.5415) (402.9892, -283.0038) (403.0834, -283.4659) (403.1796, -283.9281) (403.2779, -284.3901) (403.3782, -284.8521) (403.4805, -285.314) (403.5848, -285.7758) (403.6911, -286.2376) (403.7993, -286.6992) (403.9095, -287.1608) (404.0216, -287.6223) (404.1356, -288.0836) (404.2515, -288.5449) (404.3693, -289.006) (404.489, -289.4671) (404.6105, -289.928) (404.7339, -290.3888) (404.8591, -290.8494) (404.9861, -291.31) (405.1149, -291.7704) (405.2455, -292.2306) (405.3779, -292.6907) (405.5121, -293.1507) (405.648, -293.6105) (405.7856, -294.0701) (405.8971, -294.4377) (405.9815, -294.7134) (406.0382, -294.8971) (406.0666, -294.9889) knots 0.13851185 0.13851185 0.13851185 0.13851185 0.13851185 0.13851185 0.14285714 0.15714286 0.17142857 0.18571429 0.2 0.21428571 0.22857143 0.24285714 0.25714286 0.27142857 0.28571429 0.3 0.31428571 0.32857143 0.34285714 0.35714286 0.37142857 0.38571429 0.4 0.41428571 0.42857143 0.44285714 0.45714286 0.47142857 0.48571429 0.5 0.51428571 0.52857143 0.54285714 0.55714286 0.57142857 0.58571429 0.6 0.61428571 0.62857143 0.64285714 0.65714286 0.67142857 0.68571429 0.7 0.71428571 0.72857143 0.74285714 0.75714286 0.77142857 0.78571429 0.8 0.81428571 0.82857143 0.84285714 0.85714286 0.87142857 0.88571429 0.9 0.91428571 0.92857143 0.94285714 0.95714286 0.97142857 0.98571429 1 1 1 1 1 1
  arc A67 (406.0666, -294.9889) -> (415.7983, -296.2702) centre (452.3696, 19.1166) ccw
  spline S134 degree 5 poles (415.7983, -296.2702) (415.8495, -296.1888) (415.9518, -296.026) (416.1046, -295.7816) (416.3075, -295.4554) (416.5594, -295.047) (416.8097, -294.638) (417.0583, -294.2285) (417.3053, -293.8183) (417.5505, -293.4075) (417.7941, -292.9962) (418.036, -292.5842) (418.2762, -292.1717) (418.5146, -291.7585) (418.7513, -291.3447) (418.9862, -290.9304) (419.2193, -290.5154) (419.4507, -290.0999) (419.6802, -289.6838) (419.908, -289.267) (420.1338, -288.8497) (420.3579, -288.4318) (420.5801, -288.0133) (420.8003, -287.5942) (421.0187, -287.1745) (421.2352, -286.7542) (421.4497, -286.3334) (421.6622, -285.9119) (421.8728, -285.4898) (422.0814, -285.0672) (422.2879, -284.644) (422.4924, -284.2201) (422.6948, -283.7957) (422.8952, -283.3707) (423.0934, -282.9451) (423.2894, -282.5189) (423.4833, -282.0921) (423.675, -281.6647) (423.8645, -281.2368) (424.0517, -280.8082) (424.2366, -280.379) (424.4192, -279.9493) (424.5994, -279.5189) (424.7772, -279.088) (424.9527, -278.6564) (425.1256, -278.2242) (425.296, -277.7915) (425.4638, -277.3581) (425.6289, -276.9241) (425.7914, -276.4896) (425.9512, -276.0544) (426.1082, -275.6185) (426.2625, -275.1821) (426.4139, -274.7451) (426.5624, -274.3074) (426.7077, -273.8691) (426.8498, -273.4302) (426.9885, -272.9906) (427.1237, -272.5503) (427.2555, -272.1094) (427.3838, -271.6678) (427.4913, -271.2872) (427.5718, -270.9946) (427.627, -270.7903) (427.6579, -270.6747) (427.6651, -270.6477) knots -1 -1 -1 -1 -1 -1 -0.98571429 -0.97142857 -0.95714286 -0.94285714 -0.92857143 -0.91428571 -0.9 -0.88571429 -0.87142857 -0.85714286 -0.84285714 -0.82857143 -0.81428571 -0.8 -0.78571429 -0.77142857 -0.75714286 -0.74285714 -0.72857143 -0.71428571 -0.7 -0.68571429 -0.67142857 -0.65714286 -0.64285714 -0.62857143 -0.61428571 -0.6 -0.58571429 -0.57142857 -0.55714286 -0.54285714 -0.52857143 -0.51428571 -0.5 -0.48571429 -0.47142857 -0.45714286 -0.44285714 -0.42857143 -0.41428571 -0.4 -0.38571429 -0.37142857 -0.35714286 -0.34285714 -0.32857143 -0.31428571 -0.3 -0.28571429 -0.27142857 -0.25714286 -0.24285714 -0.22857143 -0.21428571 -0.2 -0.18571429 -0.17142857 -0.15714286 -0.14285714 -0.13851185 -0.13851185 -0.13851185 -0.13851185 -0.13851185 -0.13851185
  spline S135 degree 3 poles (429.3254, -269.474) (429.1194, -269.4576) (428.9121, -269.4815) (428.5183, -269.6075) (428.3356, -269.7084) (428.0534, -269.9457) (427.9461, -270.0684) (427.7723, -270.3419) (427.7068, -270.4911) (427.6651, -270.6477) knots 0 0 0 0 0.062015 0.062015 0.12403 0.12403 0.172638 0.172638 0.221247 0.221247 0.221247 0.221247
  arc A68 (429.3254, -269.474) -> (437.5479, -270.013) centre (452.3696, 19.1166) ccw
  spline S136 degree 3 poles (439.0408, -271.3933) (439.0141, -271.1883) (438.9476, -270.9905) (438.7426, -270.6315) (438.606, -270.4738) (438.3152, -270.247) (438.173, -270.1675) (437.8693, -270.0543) (437.7097, -270.0213) (437.5479, -270.013) knots 0 0 0 0 0.062015 0.062015 0.12403 0.12403 0.172638 0.172638 0.221247 0.221247 0.221247 0.221247
  spline S137 degree 5 poles (439.0408, -271.3933) (439.0444, -271.421) (439.06, -271.5397) (439.088, -271.7494) (439.1297, -272.05) (439.1866, -272.4414) (439.2561, -272.896) (439.3292, -273.3503) (439.4059, -273.8045) (439.486, -274.2584) (439.5696, -274.7121) (439.6564, -275.1657) (439.7465, -275.6189) (439.8395, -276.072) (439.9355, -276.5248) (440.0344, -276.9774) (440.136, -277.4297) (440.2403, -277.8818) (440.3474, -278.3336) (440.4572, -278.7852) (440.5697, -279.2365) (440.6847, -279.6875) (440.8023, -280.1383) (440.9224, -280.5888) (441.0449, -281.039) (441.1698, -281.4889) (441.2971, -281.9385) (441.4268, -282.3879) (441.5588, -282.8369) (441.693, -283.2856) (441.8295, -283.7341) (441.9683, -284.1822) (442.1093, -284.6301) (442.2524, -285.0776) (442.3977, -285.5248) (442.5451, -285.9717) (442.6947, -286.4183) (442.8463, -286.8645) (443, -287.3105) (443.1557, -287.7561) (443.3134, -288.2013) (443.4732, -288.6463) (443.6349, -289.0909) (443.7986, -289.5351) (443.9642, -289.9791) (444.1318, -290.4226) (444.3013, -290.8659) (444.4727, -291.3088) (444.6459, -291.7513) (444.8211, -292.1935) (444.9981, -292.6353) (445.1769, -293.0768) (445.3575, -293.5179) (445.54, -293.9586) (445.7242, -294.399) (445.9103, -294.839) (446.0981, -295.2787) (446.2877, -295.7179) (446.479, -296.1568) (446.672, -296.5953) (446.8667, -297.0335) (447.0632, -297.4712) (447.2217, -297.8211) (447.3414, -298.0834) (447.4215, -298.2581) (447.4617, -298.3455) knots 0.13851185 0.13851185 0.13851185 0.13851185 0.13851185 0.13851185 0.14285714 0.15714286 0.17142857 0.18571429 0.2 0.21428571 0.22857143 0.24285714 0.25714286 0.27142857 0.28571429 0.3 0.31428571 0.32857143 0.34285714 0.35714286 0.37142857 0.38571429 0.4 0.41428571 0.42857143 0.44285714 0.45714286 0.47142857 0.48571429 0.5 0.51428571 0.52857143 0.54285714 0.55714286 0.57142857 0.58571429 0.6 0.61428571 0.62857143 0.64285714 0.65714286 0.67142857 0.68571429 0.7 0.71428571 0.72857143 0.74285714 0.75714286 0.77142857 0.78571429 0.8 0.81428571 0.82857143 0.84285714 0.85714286 0.87142857 0.88571429 0.9 0.91428571 0.92857143 0.94285714 0.95714286 0.97142857 0.98571429 1 1 1 1 1 1
  arc A69 (447.4617, -298.3455) -> (457.2774, -298.3455) centre (452.3696, 19.1166) ccw
  spline S138 degree 5 poles (457.2774, -298.3455) (457.3176, -298.2581) (457.3977, -298.0834) (457.5174, -297.8211) (457.6759, -297.4712) (457.8724, -297.0335) (458.0671, -296.5953) (458.2601, -296.1568) (458.4515, -295.7179) (458.641, -295.2787) (458.8288, -294.839) (459.0149, -294.399) (459.1991, -293.9586) (459.3816, -293.5179) (459.5622, -293.0768) (459.741, -292.6353) (459.918, -292.1935) (460.0932, -291.7513) (460.2664, -291.3088) (460.4378, -290.8659) (460.6073, -290.4226) (460.7749, -289.9791) (460.9405, -289.5351) (461.1042, -289.0909) (461.2659, -288.6463) (461.4257, -288.2013) (461.5834, -287.7561) (461.7391, -287.3105) (461.8928, -286.8645) (462.0444, -286.4183) (462.194, -285.9717) (462.3414, -285.5248) (462.4867, -285.0776) (462.6298, -284.6301) (462.7708, -284.1822) (462.9096, -283.7341) (463.0461, -283.2856) (463.1803, -282.8369) (463.3123, -282.3879) (463.442, -281.9385) (463.5693, -281.4889) (463.6942, -281.039) (463.8167, -280.5888) (463.9368, -280.1383) (464.0544, -279.6875) (464.1694, -279.2365) (464.2819, -278.7852) (464.3917, -278.3336) (464.4988, -277.8818) (464.6031, -277.4297) (464.7048, -276.9774) (464.8036, -276.5248) (464.8996, -276.072) (464.9926, -275.6189) (465.0827, -275.1657) (465.1695, -274.7121) (465.2531, -274.2584) (465.3333, -273.8045) (465.4099, -273.3503) (465.483, -272.896) (465.5526, -272.4414) (465.6094, -272.05) (465.6511, -271.7494) (465.6791, -271.5397) (465.6947, -271.421) (465.6983, -271.3933) knots -1 -1 -1 -1 -1 -1 -0.98571429 -0.97142857 -0.95714286 -0.94285714 -0.92857143 -0.91428571 -0.9 -0.88571429 -0.87142857 -0.85714286 -0.84285714 -0.82857143 -0.81428571 -0.8 -0.78571429 -0.77142857 -0.75714286 -0.74285714 -0.72857143 -0.71428571 -0.7 -0.68571429 -0.67142857 -0.65714286 -0.64285714 -0.62857143 -0.61428571 -0.6 -0.58571429 -0.57142857 -0.55714286 -0.54285714 -0.52857143 -0.51428571 -0.5 -0.48571429 -0.47142857 -0.45714286 -0.44285714 -0.42857143 -0.41428571 -0.4 -0.38571429 -0.37142857 -0.35714286 -0.34285714 -0.32857143 -0.31428571 -0.3 -0.28571429 -0.27142857 -0.25714286 -0.24285714 -0.22857143 -0.21428571 -0.2 -0.18571429 -0.17142857 -0.15714286 -0.14285714 -0.13851185 -0.13851185 -0.13851185 -0.13851185 -0.13851185 -0.13851185
  spline S139 degree 3 poles (467.1912, -270.013) (466.9848, -270.0235) (466.7824, -270.0743) (466.4084, -270.2507) (466.2405, -270.3745) (465.9916, -270.6467) (465.9012, -270.7823) (465.7646, -271.0761) (465.7192, -271.2326) (465.6983, -271.3933) knots 0 0 0 0 0.062015 0.062015 0.12403 0.12403 0.172638 0.172638 0.221247 0.221247 0.221247 0.221247
  arc A70 (467.1912, -270.013) -> (475.4137, -269.474) centre (452.3696, 19.1166) ccw
  spline S140 degree 3 poles (477.074, -270.6477) (477.0208, -270.448) (476.929, -270.2605) (476.6789, -269.9314) (476.5229, -269.7928) (476.205, -269.6059) (476.0536, -269.5456) (475.7377, -269.473) (475.5752, -269.4611) (475.4137, -269.474) knots 0 0 0 0 0.062015 0.062015 0.12403 0.12403 0.172638 0.172638 0.221247 0.221247 0.221247 0.221247
  spline S141 degree 5 poles (477.074, -270.6477) (477.0812, -270.6747) (477.1121, -270.7903) (477.1673, -270.9946) (477.2478, -271.2872) (477.3553, -271.6678) (477.4836, -272.1094) (477.6154, -272.5503) (477.7506, -272.9906) (477.8893, -273.4302) (478.0314, -273.8691) (478.1767, -274.3074) (478.3252, -274.7451) (478.4766, -275.1821) (478.6309, -275.6185) (478.7879, -276.0544) (478.9477, -276.4896) (479.1102, -276.9241) (479.2753, -277.3581) (479.4431, -277.7915) (479.6135, -278.2242) (479.7864, -278.6564) (479.9619, -279.088) (480.1397, -279.5189) (480.3199, -279.9493) (480.5025, -280.379) (480.6874, -280.8082) (480.8746, -281.2368) (481.0641, -281.6647) (481.2558, -282.0921) (481.4497, -282.5189) (481.6457, -282.9451) (481.8439, -283.3707) (482.0443, -283.7957) (482.2467, -284.2201) (482.4512, -284.644) (482.6577, -285.0672) (482.8663, -285.4898) (483.0769, -285.9119) (483.2894, -286.3334) (483.5039, -286.7542) (483.7204, -287.1745) (483.9388, -287.5942) (484.1591, -288.0133) (484.3812, -288.4318) (484.6053, -288.8497) (484.8312, -289.267) (485.0589, -289.6838) (485.2884, -290.0999) (485.5198, -290.5154) (485.7529, -290.9304) (485.9878, -291.3447) (486.2245, -291.7585) (486.4629, -292.1717) (486.7031, -292.5842) (486.945, -292.9962) (487.1886, -293.4075) (487.4338, -293.8183) (487.6808, -294.2285) (487.9294, -294.638) (488.1797, -295.047) (488.4316, -295.4554) (488.6345, -295.7816) (488.7873, -296.026) (488.8896, -296.1888) (488.9408, -296.2702) knots 0.13851185 0.13851185 0.13851185 0.13851185 0.13851185 0.13851185 0.14285714 0.15714286 0.17142857 0.18571429 0.2 0.21428571 0.22857143 0.24285714 0.25714286 0.27142857 0.28571429 0.3 0.31428571 0.32857143 0.34285714 0.35714286 0.37142857 0.38571429 0.4 0.41428571 0.42857143 0.44285714 0.45714286 0.47142857 0.48571429 0.5 0.51428571 0.52857143 0.54285714 0.55714286 0.57142857 0.58571429 0.6 0.61428571 0.62857143 0.64285714 0.65714286 0.67142857 0.68571429 0.7 0.71428571 0.72857143 0.74285714 0.75714286 0.77142857 0.78571429 0.8 0.81428571 0.82857143 0.84285714 0.85714286 0.87142857 0.88571429 0.9 0.91428571 0.92857143 0.94285714 0.95714286 0.97142857 0.98571429 1 1 1 1 1 1
  arc A71 (488.9408, -296.2702) -> (498.6725, -294.9889) centre (452.3696, 19.1166) ccw